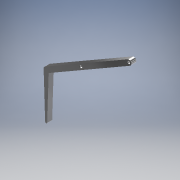
# Autodesk Inventor part: Leg Spider Crab
Saved by Autodesk Inventor 2019 (Build 230136000, 136)
## iProperties
Created: 2019-08-25
Part Number: Leg Spider Crab
Material: Aluminum 6061
Document SubType Name: Modeling
Designer: DIBYOJYOTI
Density: 2.7 g/cm^3
Appearance: Aluminum - Flat
Mass: 68.8055 g
Surface Area: 111.477 cm^2
Volume: 25.4835 cm^3
Sheet Metal Rule: Default
Author: DIBYOJYOTI
Autodesk Inventor part; units mm, degrees
ref_plane "YZ Plane" through (0, 0, 0) normal (1, 0, 0) x (0, 1, 0)
ref_plane "XZ Plane" through (0, 0, 0) normal (0, 1, 0) x (-1, 0, 0)
ref_plane "XY Plane" through (0, 0, 0) normal (0, 0, 1) x (1, 0, 0)
sketch "Sketch1" plane through (0, 0, 0) normal (0, 0, 1) x (1, 0, 0)
  circle A0 centre (134.3503, 224.3503) radius 2
  arc A1 (-3.5355, 93.5355) -> (-4.9889, 89.6672) centre (0, 90) ccw
  arc A2 (137.8858, 220.8148) -> (130.8148, 227.8858) centre (134.3503, 224.3503) ccw
  arc A3 (-1.9989, -0.0666) -> (1.9987, -0.0722) centre (0, 0) ccw
  circle A4 centre (56.5685, 146.5685) radius 2
  line L0 (-5, 90) -> (-1.9989, -0.0666)
  line L1 (130.8148, 227.8858) -> (-3.5355, 93.5355)
  line L2 (137.8858, 220.8148) -> (5.1833, 88.1122)
  line L3 (5.1833, 88.1122) -> (1.9987, -0.0722)
  dimension "d5" = 4
  dimension "d6" = 10
  dimension "d7" = 10
  dimension "d8" = 4
  dimension "d9" = 4
  dimension "d23" = 90
  dimension "d30" = 5
  dimension "d45" = 80
  dimension "d46" = 110
  dimension "d47" = 135
  constraints: 8 end point, 7 point on circle, 6 tangent, 5 centre point, 2 coincident, 1 point on line
  measures "d5" diameter of A0
  measures "d6" diameter of A1
  measures "d7" diameter of A2
  measures "d8" diameter of A3
  measures "d9" diameter of A4
  measures "d23" distance of point (0, 0) A1.centre
  measures "d30" distance from line of A4.centre L2
  measures "d45" distance of A4.centre A1.centre
  measures "d46" distance of A0.centre A4.centre
extrude "Extrusion2" add sketch "Sketch1" along normal blind 10 contours L1 A2 L2 L3 A3 L0 A1
fillet "Fillet1" radius 1 1 edges at (54.5685, 146.5685, 10)
fillet "Fillet2" radius 1 3 edges at (54.5685, 146.5685, 0) (132.3503, 224.3503, 0) (132.3503, 224.3503, 10)
equation "\"BendRadius\" = Thickness"
equation "\"BendReliefWidth\" = Thickness"
equation "\"BendReliefDepth\" = 0.5 * Thickness"
equation "\"CornerReliefSize\" = 4 * Thickness"
equation "\"MinimumRemnant\" = 2 * Thickness"
equation "\"TransitionRadius\" = BendRadius"
equation "\"JacobiRadiusSize\" = Thickness"
equation "\"GapSize\" = Thickness"
equation "\"Thickness\" = 0.5"
body "Solid2"
